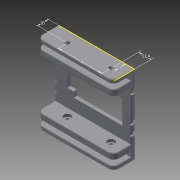
# Autodesk Inventor part: transversal
Saved by Autodesk Inventor 2015 (Build 190159000, 159)
## iProperties
Created: 2015-06-28
Part Number: transversal
Material: Genérico
Document SubType Name: Modeling
Designer: Roberto
Density: 1 g/cm^3
Appearance: Valor por defecto
Author: Roberto
Autodesk Inventor part; units mm, degrees
ref_plane "YZ Plane" through (0, 0, 0) normal (1, 0, 0) x (0, 1, 0)
ref_plane "XZ Plane" through (0, 0, 0) normal (0, 1, 0) x (-1, 0, 0)
ref_plane "XY Plane" through (0, 0, 0) normal (0, 0, 1) x (1, 0, 0)
sketch "Boceto1" plane through (0, 0, 0) normal (0, 1, 0) x (-1, 0, 0)
  line L0 (35, -36.25) -> (-35, -36.25)
  line L1 (-35, -36.25) -> (-35, 36.25)
  line L2 (-35, 36.25) -> (35, 36.25)
  line L3 (35, 36.25) -> (35, -36.25)
  line L4 (35, -36.25) -> (-35, 36.25) construction
  line L5 (-35, -36.25) -> (35, 36.25) construction
  point P0 (0, 0)
  dimension "d0" = 70
  dimension "d1" = 72.5
  constraints: 12 end point, 2 midpoint, 2 parallel, 1 horizontal, 1 perpendicular
  measures "d0" distance of L1.end L2.end
  measures "d1" distance of L2.end L0.start
extrude "Extrusión1" add sketch "Boceto1" against normal blind 3
sketch "Boceto2" plane through (0, -3, 0) normal (0, -1, 0) x (1, 0, 0)
  line L0 (-35, 36.25) -> (35, 36.25)
  line L1 (35, 36.25) -> (35, 32.25)
  line L2 (35, 32.25) -> (-35, 32.25)
  line L3 (-35, 32.25) -> (-35, 36.25)
  line L4 (-35, 28.25) -> (35, 28.25)
  line L5 (35, 28.25) -> (35, 22.25)
  line L6 (35, 22.25) -> (-35, 22.25)
  line L7 (-35, 22.25) -> (-35, 28.25)
  line L8 (-35, -32.25) -> (35, -32.25)
  line L9 (35, -32.25) -> (35, -36.25)
  line L10 (35, -36.25) -> (-35, -36.25)
  line L11 (-35, -36.25) -> (-35, -32.25)
  line L12 (-35, -22.25) -> (35, -22.25)
  line L13 (35, -22.25) -> (35, -28.25)
  line L14 (35, -28.25) -> (-35, -28.25)
  line L15 (-35, -28.25) -> (-35, -22.25)
  line L16 (-35, 36.25) -> (-35, -36.25) projected
  line L17 (35, 36.25) -> (-35, 36.25) projected
  line L18 (35, -36.25) -> (35, 36.25) projected
  line L19 (-35, -36.25) -> (35, -36.25) projected
  point P0 (0, 0)
  dimension "d4" = 4
  dimension "d5" = 4
  dimension "d6" = 6
  dimension "d7" = 4
  dimension "d8" = 4
  dimension "d9" = 6
  constraints: 32 end point, 10 collinear, 8 parallel, 4 horizontal, 4 perpendicular
  measures "d4" distance of L2.end L0.start
  measures "d5" distance between parallel lines of L2 L4
  measures "d6" distance between parallel lines of L4 L6
  measures "d7" distance between parallel lines of L8 L10
  measures "d8" distance between parallel lines of L14 L8
  measures "d9" distance between parallel lines of L12 L14
extrude "Extrusión2" add sketch "Boceto2" along normal blind 16 contours L0 L1 L2 L3 | L4 L5 L6 L7 | L12 L13 L14 L15 | L8 L9 L10 L11
sketch "Boceto3" plane through (-35, 0, 36.25) normal (0, 0, 1) x (1, 0, 0)
  line L0 (70, 0) -> (0, 0) projected
  line L1 (70, 0) -> (70, -19) projected
  point P0 (35, 0)
  point P1 (18.6, -10)
  point P2 (58.6, -10)
  dimension "d12" = 10
  dimension "d13" = 40
  dimension "d14" = 10
  dimension "d15" = 11.4
  measures "d12" distance from line of L0 point (18.6, -10)
  measures "d13" distance of point (58.6, -10) point (18.6, -10)
  measures "d14" distance from line of L0 point (58.6, -10)
  measures "d15" distance from line of point (58.6, -10) L1
sketch "Boceto4" plane through (35, -3, 22.25) normal (0, 0, -1) x (-1, 0, 0)
  point P0 (35, 3)
  point P1 (11.4, -7)
  point P2 (11.4, -7)
  point P3 (51.4, -7)
  constraints: 1 coincident
hole "Agujero1" at (-16.4, -10, 22.25) at (23.6, -10, 22.25) direction (0, 0, 1) diameter 3.6 end through all counterbore diameter 6.5 counterbore depth 2.4 clearance for "Vite intagliata a testa cilindrica ISO 1207" size "M3" standard "ISO"
sketch "Boceto5" plane through (-35, -3, -22.25) normal (0, 0, 1) x (1, 0, 0)
  point P0 (35, 3)
  point P1 (18.6, -7)
  point P2 (58.6, -7)
hole "Agujero2" at (-16.4, -10, -22.25) at (23.6, -10, -22.25) direction (0, 0, -1) diameter 3.6 end through all counterbore diameter 6.5 counterbore depth 2.4 clearance for "Vite intagliata a testa cilindrica ISO 1207" size "M3" standard "ISO"
fillet "Empalme1" radius 5 8 edges at (-35, -19, 34.25) (-35, -19, 25.25) (35, -19, 34.25) (35, -19, 25.25) (35, -19, -25.25) (35, -19, -34.25) (-35, -19, -25.25) (-35, -19, -34.25)
fillet "Empalme2" radius 1 42 edges at (-33.5355, -17.5355, -36.25) (0, -19, -36.25) (33.5355, -17.5355, -36.25) (35, -7, -36.25) (-35, -7, -36.25) (-33.5355, -17.5355, -32.25) (0, -19, -32.25) (33.5355, -17.5355, -32.25) (35, -8.5, -32.25) (-35, -8.5, -32.25) (-33.5355, -17.5355, -28.25) (0, -19, -28.25) (33.5355, -17.5355, -28.25) (35, -8.5, -28.25) (-35, -8.5, -28.25) (-33.5355, -17.5355, -22.25) (0, -19, -22.25) (33.5355, -17.5355, -22.25) (35, -8.5, -22.25) (-35, -8.5, -22.25) (-33.5355, -17.5355, 22.25) (0, -19, 22.25) (33.5355, -17.5355, 22.25) (35, -8.5, 22.25) (-35, -8.5, 22.25) (-33.5355, -17.5355, 28.25) (0, -19, 28.25) (33.5355, -17.5355, 28.25) (35, -8.5, 28.25) (-35, -8.5, 28.25) (-33.5355, -17.5355, 32.25) (0, -19, 32.25) (33.5355, -17.5355, 32.25) (35, -8.5, 32.25) (-35, -8.5, 32.25) (-33.5355, -17.5355, 36.25) (0, -19, 36.25) (33.5355, -17.5355, 36.25) (35, -7, 36.25) (-35, -7, 36.25) (-35, -3, 0) (35, -3, 0)
sketch "Boceto6" plane through (0, 0, 0) normal (0, 1, 0) x (1, 0, 0)
  line L0 (-33.5, 16.25) -> (-33.5, 12.75) projected
  line L1 (-33.5, 16.25) -> (-35, 16.25) projected
  line L2 (-35, 12.75) -> (-33.5, 12.75) projected
  line L3 (-33.5, 7.25) -> (-35, 7.25) projected
  line L4 (-33.5, 3.75) -> (-33.5, 7.25) projected
  line L5 (-35, 3.75) -> (-33.5, 3.75) projected
  line L6 (33.5, 3.75) -> (35, 3.75) projected
  line L7 (33.5, 7.25) -> (33.5, 3.75) projected
  line L8 (35, 7.25) -> (33.5, 7.25) projected
  line L9 (33.5, 12.75) -> (35, 12.75) projected
  line L10 (33.5, 16.25) -> (33.5, 12.75) projected
  line L11 (35, 16.25) -> (33.5, 16.25) projected
  line L12 (-35, -35.25) -> (-35, 35.25) projected
  line L13 (35, 35.25) -> (35, -35.25) projected
  line L14 (-33.5, -16.65) -> (-35, -16.65) projected
  line L15 (-33.5, -20.15) -> (-33.5, -16.65) projected
  line L16 (-35, -20.15) -> (-33.5, -20.15) projected
  line L17 (33.5, -20.25) -> (33.5, -16.75) projected
  line L18 (35, -16.75) -> (33.5, -16.75) projected
  line L19 (33.5, -20.25) -> (35, -20.25) projected
  point P0 (0, 0)
extrude "Extrusión3" cut sketch "Boceto6" against normal up to next
sketch "Boceto8" plane through (0, -3, 0) normal (0, -1, 0) x (1, 0, 0)
  line L0 (25.75, 9.35) -> (25.75, -10.25) projected
  line L1 (25.75, 9.35) -> (-15.15, 9.35) projected
  line L2 (-15.15, 9.35) -> (-15.15, 3.05) projected
  line L3 (-15.15, 3.05) -> (-21.15, 3.05) projected
  line L4 (-21.15, -3.95) -> (-21.15, 3.05) projected
  line L5 (-15.15, -3.95) -> (-21.15, -3.95) projected
  line L6 (-15.15, -3.95) -> (-15.15, -10.25) projected
  line L7 (25.75, -10.25) -> (-15.15, -10.25) projected
  line L8 (25.75, 9.35) -> (25.75, -10.25) projected
  line L9 (26.75, 9.85) -> (-16.15, 9.85)
  line L10 (-16.15, 9.85) -> (-16.15, 4.05)
  line L11 (-16.15, 4.05) -> (-22.15, 4.05)
  line L12 (-22.15, 4.05) -> (-22.15, -4.95)
  line L13 (-22.15, -4.95) -> (-16.15, -4.95)
  line L14 (-16.15, -4.95) -> (-16.15, -10.75)
  line L15 (-16.15, -10.75) -> (26.75, -10.75)
  line L16 (26.75, 9.85) -> (26.75, -10.75)
  point P0 (0, 0)
  dimension "d34" = 0.5
  dimension "d36" = 1
  dimension "d37" = 0.5
  dimension "d38" = 1
  constraints: 16 end point, 1 vertical, 4 other
  measures "d34" distance between parallel lines of L9 L1
  measures "d36" distance between parallel lines of L0 L16
  measures "d37" distance between parallel lines of L15 L7
  measures "d38" distance between parallel lines of L14 L6
ref_plane "Plano de trabajo1" through (-35, 0, -36.25) normal (0, -1, 0) x (1, 0, 0)
extrude "Extrusión4" cut sketch "Boceto8" against normal up to surface (3 mm away) contours L0 L7 L6 L5 L4 L3 L2 L1 | L16 L15 L14 L13 L12 L11 L10 L9
sketch "Boceto10" plane through (0, -3, 0) normal (0, -1, 0) x (1, 0, 0)
  arc A0 (26.1843, -16.25) -> (23.8157, -16.25) centre (25, -15.25) ccw
  circle A1 centre (25, 14.25) radius 1.55
  circle A2 centre (-29, 18.25) radius 1.55
  circle A3 centre (-29, -17.25) radius 1.55
  point P0 (0, 0)
  constraints: 4 centre point, 4 coincident, 2 point on circle, 10 other
hole "Agujero3" at (25, -3, 14.25) at (25, -3, -15.25) at (-29, -3, -17.25) at (-29, -3, 18.25) direction (0, 1, 0) diameter 3.1 end through all
